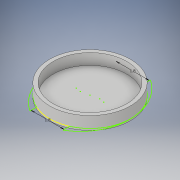
# Autodesk Inventor part: watchBodyOne
Saved by Autodesk Inventor 2019 (Build 230136000, 136)
## iProperties
Created: 2019-10-08
Part Number: watchBodyOne
Material: Generic
Document SubType Name: Modeling
Designer: Derek
Density: 1 g/cm^3
Appearance: Default
Author: Derek
Autodesk Inventor part; units mm, degrees
ref_plane "YZ Plane" through (0, 0, 0) normal (1, 0, 0) x (0, 1, 0)
ref_plane "XZ Plane" through (0, 0, 0) normal (0, 1, 0) x (-1, 0, 0)
ref_plane "XY Plane" through (0, 0, 0) normal (0, 0, 1) x (1, 0, 0)
sketch "Sketch1" plane through (0, 0, 0) normal (0, 1, 0) x (-1, 0, 0)
  circle A0 centre (0, 0) radius 22
  arc A1 (-13.7238, -17.1947) -> (13.7238, -17.1947) centre (0, 0) ccw
  dimension "d0" = 44
  dimension "d11" = 13.7238
  constraints: 4 point on circle, 2 centre point, 1 coincident, 1 concentric
  measures "d0" diameter of A0
  measures "d11" horizontal distance of point (0, 0) A0.start
extrude "Main Base" add sketch "Sketch1" along normal blind 7
sketch "Sketch5" plane through (0, 7, 0) normal (0, 1, 0) x (1, 0, 0)
  circle A0 centre (0, 0) radius 20
  dimension "d8" = 40
  constraints: 1 centre point, 1 coincident
  measures "d8" diameter of A0
extrude "Hole" cut sketch "Sketch5" against normal blind 6
sketch "Sketch16" plane through (0, 1, 0) normal (0, 1, 0) x (1, 0, 0)
  circle A0 centre (0, 0) radius 22 projected
  line L0 (9.0259, 20.0632) -> (9.0259, 23.7188)
  line L1 (-8.9741, 20.0864) -> (-8.9741, 23.7188)
  arc A1 (22, 0) -> (9.0259, 23.7188) centre (-6.9981, -0.4541) ccw
  arc A2 (8.9741, -23.7188) -> (22, 0) centre (-4.3501, -0.9652) ccw
  arc A3 (-22, 0) -> (-9.0259, -20.0632) centre (0, 0) ccw
  arc A4 (8.9741, -20.0864) -> (22, 0) centre (0, 0) ccw
  line L2 (-9.0259, -20.0632) -> (-9.0259, -23.7188)
  line L3 (8.9741, -20.0864) -> (8.9741, -23.7188)
  arc A5 (-22, 0) -> (-9.0259, -23.7188) centre (6.9981, 0.4541) ccw
  arc A6 (-8.9741, 23.7188) -> (-22, 0) centre (4.3501, 0.9652) ccw
  arc A7 (-22, 0) -> (-9.0259, -20.0632) centre (0, 0) ccw
  arc A8 (8.9741, -20.0864) -> (22, 0) centre (0, 0) ccw
  arc A9 (-8.9741, 20.0864) -> (-22, 0) centre (0, 0) ccw
  arc A10 (22, 0) -> (9.0259, 20.0632) centre (0, 0) ccw
  arc A11 (8.9741, -20.0864) -> (22, 0) centre (0, 0) ccw
  arc A12 (-22, 0) -> (-9.0259, -20.0632) centre (0, 0) ccw
  dimension "d44" = 18
  dimension "d45" = 18
  constraints: 24 point on circle, 12 centre point, 8 end point, 4 concentric, 2 vertical, 1 horizontal alignment, 5 other
  measures "d44" distance between parallel lines of L1 L0
  measures "d45" distance between parallel lines of L3 L2
body "Solid1"
